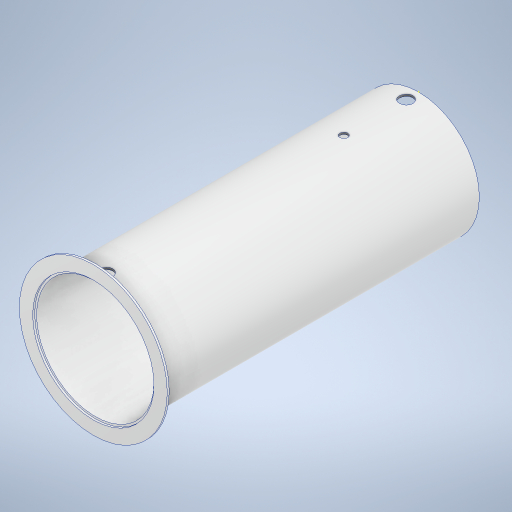
# Autodesk Inventor part: stainless steel outer wall
Saved by Autodesk Inventor 2023 (Build 270158000, 158)
## iProperties
Created: 2022-09-19
Part Number: stainless steel outer wall
Material: Aluminum 6061
Document SubType Name: Modeling
Designer: station
Density: 2.7 g/cm^3
Appearance: Aluminum - Flat
Author: station
Autodesk Inventor part; units mm, degrees
ref_plane "YZ Plane" through (0, 0, 0) normal (1, 0, 0) x (0, 1, 0)
ref_plane "XY Plane" through (0, 0, 0) normal (0, 0, 1) x (1, 0, 0)
sketch "Sketch1" plane through (0, 0, 0) normal (0, 0, 1) x (1, 0, 0)
  circle A0 centre (0, 0) radius 59.5
  circle A1 centre (0, 0) radius 61.5
  dimension "d0" = 119
  dimension "d1" = 123
  constraints: 2 centre point, 2 coincident
  measures "d0" diameter of A0
  measures "d1" diameter of A1
extrude "Extrusion1" add sketch "Sketch1" along normal blind 328
ref_plane "Work Plane1" through (0, 61.5, 0) normal (0, 1, 0) x (-1, 0, 0)
sketch "Sketch2" plane through (0, 61.5, 0) normal (0, 1, 0) x (-1, 0, 0)
  line L0 (61.5, 0) -> (-61.5, 0) projected
  line L1 (0, 0) -> (0, 4)
  line L2 (0, 4) -> (0, 6)
  circle A0 centre (0, 12.858) radius 6.858
  dimension "d6" = 4
  dimension "d7" = 2
  dimension "d8" = 13.716
  dimension "d9" = 6.858
  constraints: 4 end point, 1 centre point, 1 point on line, 1 vertical
  measures "d6" distance of L1.start L1.end
  measures "d7" distance of L1.end L2.end
  measures "d8" diameter of A0
  measures "d9" distance of A0.centre L2.end
extrude "Extrusion2" cut sketch "Sketch2" against normal blind 23
sketch "Sketch3" plane through (0, 61.5, 0) normal (0, 1, 0) x (-1, 0, 0)
  line L0 (0, 0) -> (0, 328) construction
  line L1 (-59.5, 328) -> (59.5, 328) projected
  line L2 (0, 328) -> (0, 320) construction
  circle A0 centre (0, 317.142) radius 6.858
  point P0 (0, 324)
  dimension "d12" = 8
  dimension "d13" = 13.716
  dimension "d14" = 6.858
  constraints: 4 end point, 2 midpoint, 2 point on line, 1 centre point
  measures "d12" distance of L0.end L2.end
  measures "d13" diameter of A0
  measures "d14" distance of A0.centre point (0, 324)
extrude "Extrusion3" cut sketch "Sketch3" against normal blind 3
thread "Thread1" size "M14x1.25" class "6H" standard "ANSI Metric M Profile" full length
thread "Thread2" size "M14x1.25" class "6H" standard "ANSI Metric M Profile" full length
sketch "Sketch4" plane through (0, 61.5, 0) normal (0, 1, 0) x (-1, 0, 0)
  point P0 (0, 0)
sketch "Sketch5" plane through (0, 61.5, 0) normal (0, 1, 0) x (-1, 0, 0)
  line L0 (0, 0) -> (0, 76) construction
  circle A0 centre (0, 76) radius 4
  dimension "d21" = 76
  dimension "d22" = 8
  constraints: 2 end point, 1 centre point, 1 coincident, 1 vertical
  measures "d21" distance of L0.start L0.end
  measures "d22" diameter of A0
extrude "Extrusion4" cut sketch "Sketch5" against normal through all
thread "Thread3" size "M8x1.25" class "6H" standard "ANSI Metric M Profile" full length
thread "Thread4" size "M8x1.25" class "6H" standard "ANSI Metric M Profile" full length
sketch "Sketch6" plane through (0, 0, 328) normal (0, 0, 1) x (1, 0, 0)
  circle A0 centre (0, 0) radius 75
  circle A1 centre (0, 0) radius 61.5
  dimension "d29" = 150
  dimension "d30" = 123
  constraints: 2 centre point, 2 coincident
  measures "d29" diameter of A0
  measures "d30" diameter of A1
extrude "Extrusion5" add sketch "Sketch6" along normal blind 2
body "Solid1"
